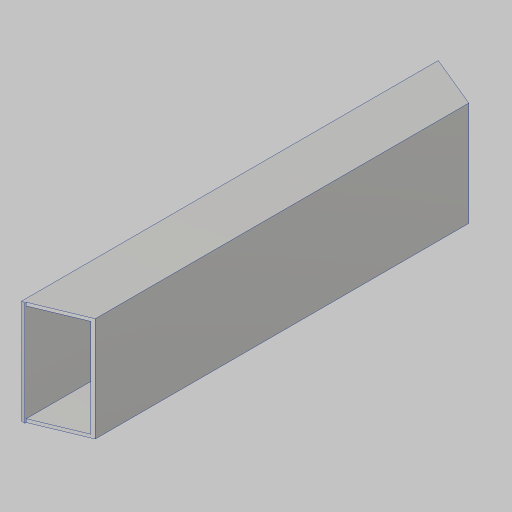
# Autodesk Inventor part: CL3-002
Saved by Autodesk Inventor 2023.5 (Build 275446000, 446)
## iProperties
RuleStatus: InUse
Created: 2025-01-28
Part Number: CL3-002
Material: Aluminum 6061
Document SubType Name: Modeling
Designer: slick
Mass: 304.185 g
Surface Area: 718.547 cm^2
Volume: 112.661 cm^3
Density: 2.7 g/cm^3
Appearance: Aluminum - Flat
AfterDocNew0: SHOW
AfterDocOpen0: SHOW
Author: slick
Autodesk Inventor part; units mm, degrees
ref_plane "YZ Plane" through (0, 0, 0) normal (1, 0, 0) x (0, 1, 0)
ref_plane "XZ Plane" through (0, 0, 0) normal (0, 1, 0) x (-1, 0, 0)
ref_plane "XY Plane" through (0, 0, 0) normal (0, 0, 1) x (1, 0, 0)
sketch "Sketch1" plane through (0, 0, 0) normal (0, 0, 1) x (1, 0, 0)
  line L0 (-12.7, -25.4) -> (12.7, -25.4)
  line L1 (12.7, -25.4) -> (12.7, 25.4)
  line L2 (12.7, 25.4) -> (-12.7, 25.4)
  line L3 (-12.7, 25.4) -> (-12.7, -25.4)
  line L4 (-12.7, -25.4) -> (12.7, 25.4) construction
  line L5 (12.7, -25.4) -> (-12.7, 25.4) construction
  line L6 (-11.1125, 23.8125) -> (11.1125, 23.8125)
  line L7 (11.1125, 23.8125) -> (11.1125, -23.8125)
  line L8 (11.1125, -23.8125) -> (-11.1125, -23.8125)
  line L9 (-11.1125, -23.8125) -> (-11.1125, 23.8125)
  point P0 (0, 0)
  dimension "width" = 25.4
  dimension "height" = 50.8
  dimension "thickness" = 1.5875
  constraints: 20 end point, 4 parallel, 2 midpoint, 2 perpendicular, 1 horizontal, 3 other
  measures "width" distance of L2.end L1.end
  measures "height" distance of L1.end L0.end
  measures "thickness" distance between parallel lines of L2 L6
extrude "Extrusion1" add sketch "Sketch1" along normal mid plane 203.2
sketch "Sketch2" plane through (-12.7, 25.4, 101.6) normal (0, 1, 0) x (1, 0, 0)
  line L0 (0, 203.2) -> (0, 0) projected
  line L1 (25.4, 0) -> (0, 0) projected
  line L2 (25.4, 203.2) -> (25.4, 0) projected
  line L3 (0, 203.2) -> (25.4, 203.2) projected
  line L4 (1.5875, 0) -> (23.8125, 0) projected
  line L5 (1.5875, 203.2) -> (1.5875, 0) projected
  line L6 (25.4, 203.2) -> (25.4, 0) projected
  line L7 (0, 0) -> (25.4, 0) construction
  line L8 (0, 0) -> (25.4, 10.521)
  line L9 (25.4, 203.2) -> (25.4, 0) construction
  point P0 (12.7, 101.6)
  point P1 (1.5875, 0.6576)
  dimension "d12" = 22.5
  constraints: 2 end point, 1 point on line
  measures "d12" angle of L1 L8
extrude "Extrusion2" cut sketch "Sketch2" against normal through all contours L5 L8 L2 L1
sketch "Sketch3" plane through (-12.7, -25.4, -101.6) normal (0, -1, 0) x (1, 0, 0)
  line L0 (0, 203.2) -> (0, 0) projected
  line L1 (25.4, 0) -> (0, 0) projected
  line L2 (25.4, 0) -> (25.4, 192.679) projected
  line L3 (0, 203.2) -> (0, 0) projected
  line L4 (0, 0) -> (25.4, 10.521)
  line L5 (25.4, 0) -> (25.4, 203.2) projected
  line L6 (0, 203.2) -> (1.5875, 203.2) projected
  line L7 (25.4, 192.679) -> (1.5875, 202.5424) projected
  line L8 (1.5875, 202.5424) -> (1.5875, 203.2) projected
  point P0 (12.7, 101.6)
  point P1 (0, 192.679)
  point P2 (25.4, 10.521)
  dimension "d11" = 67.5
  constraints: 2 end point, 1 point on line
  measures "d11" angle of L0 L4
extrude "Extrusion3" cut sketch "Sketch3" against normal through all contours L4 L2 L1
body "Solid1"
